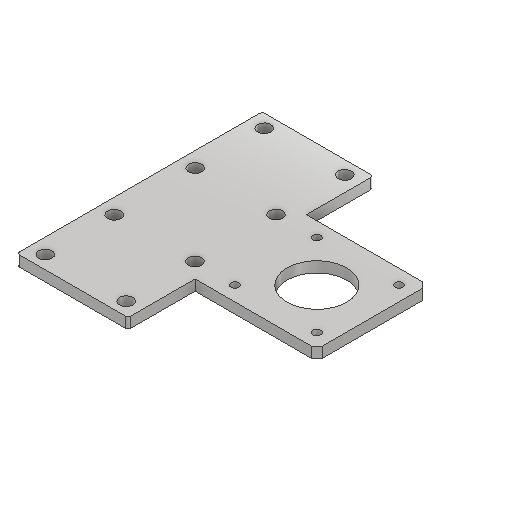
# Autodesk Inventor part: LC_ALU_4mm_X_End_Motor_Side
Saved by Autodesk Inventor 2026.1 (Build 301233000, 233)
## iProperties
Created: 2017-05-25
Part Number: LC_ALU_4mm_X_End_Motor_Side
Material: Ogólny
Document SubType Name: Modeling
Designer: Andrzej
Density: 1 g/cm^3
Appearance: Aluminium - ciemne
Mass: 20.9335 g
Surface Area: 128.315 cm^2
Volume: 20.9335 cm^3
Author: Andrzej
Autodesk Inventor part; units mm, degrees
ref_plane "YZ Plane" through (0, 0, 0) normal (1, 0, 0) x (0, 1, 0)
ref_plane "XZ Plane" through (0, 0, 0) normal (0, 1, 0) x (-1, 0, 0)
ref_plane "XY Plane" through (0, 0, 0) normal (0, 0, 1) x (1, 0, 0)
sketch "Szkic1" plane through (0, 0, 0) normal (0, 0, 1) x (1, 0, 0)
  line L0 (-10.2233, 17.3341) -> (-10.2233, -75.2659)
  line L1 (-10.2233, -75.2659) -> (31.7767, -75.2659)
  line L2 (-10.2233, 17.3341) -> (31.7767, 17.3341)
  line L3 (31.7767, 17.3341) -> (31.7767, -7.9659)
  line L4 (31.7767, -75.2659) -> (31.7767, -49.9659)
  line L5 (31.7767, -49.9659) -> (77.7767, -49.9659)
  line L6 (77.7767, -49.9659) -> (77.7767, -7.9659)
  line L7 (77.7767, -7.9659) -> (31.7767, -7.9659)
  point P0 (0, 0)
  point P1 (41.2767, -13.4659)
  point P2 (72.2767, -13.4659)
  point P3 (41.2767, -44.4659)
  point P4 (72.2767, -44.4659)
  point P5 (56.7767, -28.9659)
  point P6 (-4.4733, 12.3341)
  point P7 (26.0267, 12.3341)
  point P8 (-4.4733, -13.6659)
  point P9 (26.0267, -13.6659)
  point P10 (-4.4733, -44.2659)
  point P11 (26.0267, -44.2659)
  point P12 (-4.4733, -70.2659)
  point P13 (26.0267, -70.2659)
  dimension "d0" = 92.6
  dimension "d1" = 42
  dimension "d2" = 42
  dimension "d3" = 46
  dimension "d4" = 25.3
  dimension "d11" = 15.5
  dimension "d12" = 15.5
  dimension "d14" = 15.5
  dimension "d15" = 15.5
  dimension "d16" = 15.5
  dimension "d17" = 15.5
  dimension "d18" = 15.5
  dimension "d19" = 15.5
  dimension "d20" = 21
  dimension "d21" = 21
  dimension "d39" = 5
  dimension "d40" = 5
  dimension "d41" = 5
  dimension "d42" = 5
  dimension "d43" = 5.75
  dimension "d44" = 5.75
  dimension "d45" = 42
  dimension "d46" = 5.75
  dimension "d47" = 5.75
  dimension "d48" = 5.75
  dimension "d49" = 5.75
  dimension "d50" = 25.3
  dimension "d51" = 5.75
  dimension "d52" = 5.75
  dimension "d60" = 26
  dimension "d61" = 26
  dimension "d62" = 26
  dimension "d63" = 26
  constraints: 16 end point, 3 perpendicular, 3 vertical, 2 horizontal
  measures "d0" distance of L0.start L0.end
  measures "d1" distance of L0.end L1.end
  measures "d2" distance between parallel lines of L5 L7
  measures "d3" distance of L6.end L3.end
  measures "d4" distance between parallel lines of L2 L7
  measures "d11" horizontal distance of point (56.777, -28.966) point (41.277, -44.466)
  measures "d12" horizontal distance of point (56.777, -28.966) point (41.277, -44.466)
  measures "d14" horizontal distance of point (56.777, -28.966) point (41.277, -13.466)
  measures "d15" horizontal distance of point (56.777, -28.966) point (41.277, -13.466)
  measures "d16" horizontal distance of point (72.277, -13.466) point (56.777, -28.966)
  measures "d17" horizontal distance of point (56.777, -28.966) point (72.277, -13.466)
  measures "d18" horizontal distance of point (56.777, -28.966) point (72.277, -44.466)
  measures "d19" horizontal distance of point (56.777, -28.966) point (72.277, -44.466)
  measures "d20" distance from line of L7 point (56.777, -28.966)
  measures "d21" distance from line of L6 point (56.777, -28.966)
  measures "d39" distance from line of L2 point (-4.473, 12.334)
  measures "d40" distance from line of L2 point (26.027, 12.334)
  measures "d41" distance from line of L1 point (-4.473, -70.266)
  measures "d42" distance from line of L1 point (26.027, -70.266)
  measures "d43" distance from line of L0 point (-4.473, 12.334)
  measures "d44" distance from line of L3 point (26.027, 12.334)
  measures "d45" distance between parallel lines of L0 L3
  measures "d46" distance from line of L3 point (26.027, -13.666)
  measures "d47" distance from line of L0 point (-4.473, -13.666)
  measures "d48" distance from line of L0 point (-4.473, -44.266)
  measures "d49" distance from line of L0 point (-4.473, -70.266)
  measures "d50" distance of L1.end L4.end
  measures "d51" distance from line of L4 point (26.027, -70.266)
  measures "d52" distance from line of L4 point (26.027, -44.266)
  measures "d60" distance of point (-4.473, 12.334) point (-4.473, -13.666)
  measures "d61" distance of point (26.027, 12.334) point (26.027, -13.666)
  measures "d62" distance of point (26.027, -70.266) point (26.027, -44.266)
  measures "d63" distance of point (-4.473, -70.266) point (-4.473, -44.266)
extrude "Wyciągnięcie proste1" add sketch "Szkic1" along normal blind 4
hole "Otwór1" at (41.2767, -13.4659, 0) at (72.2767, -13.4659, 0) at (41.2767, -44.4659, 0) at (72.2767, -44.4659, 0) direction (0, 0, 1) diameter 3 end through all
hole "Otwór2" at (56.7767, -28.9659, 0) direction (0, 0, 1) diameter 22.5 end through all
chamfer "Faza1" distance 2 angle 45 2 edges at (77.7767, -7.9659, 2) (77.7767, -49.9659, 2)
hole "Otwór3" at (-4.4733, 12.3341, 0) at (26.0267, 12.3341, 0) at (-4.4733, -13.6659, 0) at (26.0267, -13.6659, 0) at (-4.4733, -44.2659, 0) at (26.0267, -44.2659, 0) at (-4.4733, -70.2659, 0) at (26.0267, -70.2659, 0) direction (0, 0, 1) diameter 5 end through all
fillet "Zaokrąglenie1" radius 1 4 edges at (31.7767, 17.3341, 2) (-10.2233, 17.3341, 2) (31.7767, -75.2659, 2) (-10.2233, -75.2659, 2)
equation "\"d4\" = -0.5 * d2 + 0.5 * d0"
equation "\"d11\" = 0.5 * d9"
equation "\"d12\" = d11"
equation "\"d14\" = d11"
equation "\"d21\" = d20"
equation "\"d39\" = d41"
equation "\"d40\" = d41"
equation "\"d42\" = d41"
equation "\"d44\" = d43"
equation "\"d45\" = d1"
equation "\"d46\" = d43"
equation "\"d47\" = d43"
equation "\"d48\" = d43"
equation "\"d49\" = d43"
equation "\"d51\" = d43"
equation "\"d52\" = d43"
equation "\"d9\" = 31"
